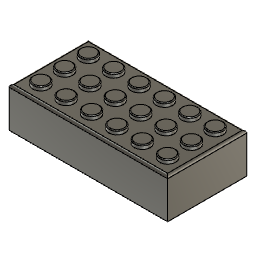
lego block v2 (Autodesk Fusion 360 design; units mm, degrees)
Autodesk Fusion 360 part; units mm, degrees
sketch "Sketch1" plane through (0, 0, 0) normal (0, 0, 1) x (1, 0, 0) in component "Lego block"
  line L0 (-100, 50) -> (100, 50)
  line L1 (100, 50) -> (100, -50)
  line L2 (100, -50) -> (-100, -50)
  line L3 (-100, -50) -> (-100, 50)
  line L4 (-100, 50) -> (100, -50) construction
  line L5 (100, 50) -> (-100, -50) construction
  dimension "d1" = 200
  constraint horizontal L0
  constraint perpendicular L0 L1
  constraint parallel L0 L2
  constraint parallel L1 L3
  constraint coincident L4 origin
  constraint coincident L5 origin
  measures "d1" distance of L1.end L2.end
extrude "Extrude1" add sketch "Sketch1" along normal blind 50 in component "Lego block"
sketch "Sketch2" plane through (0, 0, 50) normal (0, 0, 1) x (-1, 0, 0) in component "Lego block"
  line L0 (100, 50) -> (-100, 50)
  line L1 (-100, 50) -> (-100, -50)
  line L2 (-100, -50) -> (100, -50)
  line L3 (100, -50) -> (100, 50)
  circle A0 centre (-80, -30) radius 10
  circle A1 centre (-48, -30) radius 10
  circle A2 centre (-16, -30) radius 10
  circle A3 centre (16, -30) radius 10
  circle A4 centre (48, -30) radius 10
  circle A5 centre (80, -30) radius 10
  circle A6 centre (-80, 0) radius 10
  circle A7 centre (-48, 0) radius 10
  circle A8 centre (-16, 0) radius 10
  circle A9 centre (16, 0) radius 10
  circle A10 centre (48, 0) radius 10
  circle A11 centre (80, 0) radius 10
  circle A12 centre (-80, 30) radius 10
  circle A13 centre (-48, 30) radius 10
  circle A14 centre (-16, 30) radius 10
  circle A15 centre (16, 30) radius 10
  circle A16 centre (48, 30) radius 10
  circle A17 centre (80, 30) radius 10
  dimension "d4" = 20
  dimension "d5" = 20
  dimension "d6" = 20
  dimension "d9" = 160
  dimension "d10" = 60
  measures "d4" diameter of A0
  measures "d5" distance of L2 A0.centre
  measures "d6" distance of L1 A0.centre
extrude "Extrude2" add sketch "Sketch2" along normal blind 5 contours A0 | A1 | A2 | A3 | A4 | A5 | A6 | A7 | A8 | A9 | A10 | A11 | A12 | A13 | A14 | A15 | A16 | A17 in component "Lego block"
fillet "Fillet1" radius 1 18 edges at (-6.6767, 33.6162, 55) (-38.6767, 33.6162, 55) (-70.6767, 33.6162, 55) (25.3233, 33.6162, 55) (57.3233, 33.6162, 55) (89.3233, 33.6162, 55) (89.3233, 3.6162, 55) (57.3233, 3.6162, 55) (25.3233, 3.6162, 55) (-6.6767, 3.6162, 55) (-38.6767, 3.6162, 55) (-70.6767, 3.6162, 55) (-70.6767, -26.3838, 55) (-38.6767, -26.3838, 55) (-6.6767, -26.3838, 55) (25.3233, -26.3838, 55) (57.3233, -26.3838, 55) (89.3233, -26.3838, 55) in component "Lego block"
fillet "Fillet2" radius 3 4 edges at (0, 50, 50) (100, 0, 50) (-100, 0, 50) (0, -50, 50) in component "Lego block"
shell "Shell1" thickness 2 removed faces 1 at (-33.3333, 16.6667, 0) in component "Lego block"
sketch "Sketch3" plane through (0, 0, 48) normal (0, 0, -1) x (1, 0, 0) in component "Lego block"
  circle A0 centre (-16, -30) radius 8
  circle A1 centre (-80, 0) radius 8
  circle A2 centre (48, 0) radius 8
  circle A3 centre (16, 30) radius 8
  circle A4 centre (-80, 30) radius 8
  circle A5 centre (48, 30) radius 8
  circle A6 centre (-16, 0) radius 8
  circle A7 centre (80, -30) radius 8
  circle A8 centre (-48, -30) radius 8
  circle A9 centre (16, -30) radius 8
  circle A10 centre (-48, 0) radius 8
  circle A11 centre (80, 0) radius 8
  circle A12 centre (-16, 30) radius 8
  circle A13 centre (-48, 30) radius 8
  circle A14 centre (80, 30) radius 8
  circle A15 centre (16, 0) radius 8
  circle A16 centre (48, -30) radius 8
  circle A17 centre (-80, -30) radius 8
  line L0 (97, 47) -> (-97, 47)
  line L1 (-97, 47) -> (-97, -47)
  line L2 (-97, -47) -> (97, -47)
  line L3 (97, -47) -> (97, 47)
extrude "Extrude3" add sketch "Sketch3" along normal blind 1 contours A0 | A1 | A2 | A3 | A4 | A5 | A6 | A7 | A8 | A9 | A10 | A11 | A12 | A13 | A14 | A15 | A16 | A17 | L0 L1 L2 L3 in component "Lego block"
sketch "Sketch4" plane through (0, 0, 0) normal (0, 0, 1) x (1, 0, 0) in component "Lego block"
  circle A0 centre (60, 0) radius 13.3865
  circle A1 centre (60, 0) radius 18.3865
  circle A2 centre (0, 0) radius 13.3865
  circle A3 centre (0, 0) radius 18.3865
  circle A4 centre (-62.4, -0.4525) radius 13.3865
  circle A5 centre (-62.4, -0.4525) radius 18.3865
  circle A6 centre (60, 0) radius 13.3865
  circle A7 centre (60, 0) radius 18.3865
  point P0 (60, 0)
  point P1 (60, 0)
  dimension "d20" = 5
  dimension "d21" = 5
  dimension "d22" = 5
  dimension "d23" = 5
extrude "Extrude4" add sketch "Sketch4" along normal up to near side of body 1 in component "Lego block"
component "Lego block" placed x (1, 0, 0) y (0, 1, 0) z (0, 0, 1) at (0, 0, 0)
